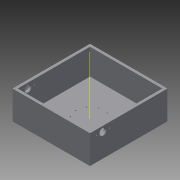
# Autodesk Inventor part: locomotion box
Saved by Autodesk Inventor 2015 (Build 190159000, 159)
## iProperties
Created: 2014-10-11
Part Number: locomotion box
Material: Generic
Document SubType Name: Modeling
Designer: ericd_000
Density: 1 g/cm^3
Appearance: Default
Author: ericd_000
Autodesk Inventor part; units mm, degrees
ref_plane "YZ Plane" through (0, 0, 0) normal (1, 0, 0) x (0, 1, 0)
ref_plane "XZ Plane" through (0, 0, 0) normal (0, 1, 0) x (-1, 0, 0)
ref_plane "XY Plane" through (0, 0, 0) normal (0, 0, 1) x (1, 0, 0)
sketch "Sketch1" plane through (0, 0, 0) normal (0, 0, 1) x (1, 0, 0)
  line L0 (-150, 150) -> (150, 150)
  line L1 (150, 150) -> (150, -150)
  line L2 (150, -150) -> (-150, -150)
  line L3 (-150, -150) -> (-150, 150)
  point P0 (0, 0)
  point P1 (150, 0)
  point P2 (0, 150)
  dimension "d0" = 300
  dimension "d1" = 300
  constraints: 8 end point, 2 midpoint, 2 parallel, 1 horizontal, 1 horizontal alignment, 1 perpendicular, 1 vertical alignment
  measures "d0" distance of L0.start L0.end
  measures "d1" distance of L0.end L1.end
extrude "Extrusion1" add sketch "Sketch1" along normal blind 10
sketch "Sketch2" plane through (0, 0, 10) normal (0, 0, 1) x (1, 0, 0)
  line L0 (-150, 150) -> (150, 150)
  line L1 (150, 150) -> (150, -150)
  line L2 (150, -150) -> (-150, -150)
  line L3 (-150, -150) -> (-150, 150)
  line L4 (140, 140) -> (-140, 140)
  line L5 (-140, 140) -> (-140, -140)
  line L6 (-140, -140) -> (140, -140)
  line L7 (140, -140) -> (140, 140)
  point P0 (0, 0)
  dimension "d4" = 10
  constraints: 16 end point, 4 parallel, 2 perpendicular, 1 horizontal, 3 other
  measures "d4" distance between parallel lines of L3 L5
extrude "Extrusion2" add sketch "Sketch2" along normal blind 100
sketch "Sketch3" plane through (-150, -150, 0) normal (-1, 0, 0) x (0, 0, 1)
  circle A0 centre (60, 250) radius 12.5
  circle A1 centre (90, 50) radius 13.3073
  line L0 (0, 300) -> (110, 300) projected
  line L1 (0, 0) -> (110, 0) projected
  line L2 (110, 300) -> (110, 0) projected
  point P0 (0, 150)
  dimension "d7" = 25
  dimension "d8" = 50
  dimension "d9" = 50
  dimension "d10" = 20
  dimension "d11" = 50
  constraints: 2 centre point
  measures "d7" diameter of A0
  measures "d8" distance from line of L0 A0.centre
  measures "d9" distance from line of L1 A1.centre
  measures "d10" distance from line of L2 A1.centre
  measures "d11" distance from line of L2 A0.centre
sketch "Sketch6" plane through (0, 0, 0) normal (0, 0, -1) x (-1, 0, 0)
  circle A0 centre (0, 0) radius 59.25
  dimension "d21" = 118.5
  constraints: 1 centre point, 1 coincident
  measures "d21" diameter of A0
extrude "Extrusion6" cut sketch "Sketch6" against normal blind 5
sketch "Sketch7" plane through (0, 0, 5) normal (0, 0, -1) x (-1, 0, 0)
  circle A0 centre (42.997, -32.6689) radius 2
  line L0 (42.997, -32.6689) -> (0, 0) construction
  dimension "d24" = 54
  dimension "d25" = 4
  constraints: 2 end point, 1 centre point
  measures "d24" distance of L0.start L0.end
  measures "d25" diameter of A0
extrude "Extrusion7" cut sketch "Sketch7" against normal up to surface (5 mm away)
pattern_circular "Circular Pattern1" count 10 over 360 about axis through (0, 0, 5) along (0, 0, 1) of "Extrusion7"
extrude "Extrusion8" cut sketch "Sketch3" against normal blind 10 contours A1
sketch "Sketch8" plane through (-150, -150, 0) normal (-1, 0, 0) x (0, 0, 1)
  circle A0 centre (90, 75.4) radius 2.05
  circle A1 centre (90, 24.6) radius 2.05
  line L0 (90, 24.6) -> (90, 75.4) construction
  line L1 (0, 0) -> (0, 300) construction
  circle A2 centre (90, 50) radius 13.3073 construction
  circle A3 centre (90, 50) radius 13.3073 construction
  point P0 (0, 150)
  dimension "d33" = 4.1
  dimension "d34" = 4.1
  dimension "d35" = 50.8
  dimension "d37" = 0
  constraints: 3 centre point, 2 end point, 1 coincident, 1 concentric, 1 midpoint, 1 parallel
  measures "d33" diameter of A0
  measures "d34" diameter of A1
  measures "d35" distance of L0.end L0.start
  measures "d37" radial gap between concentric circles of A2 A3
extrude "Extrusion9" cut sketch "Sketch8" against normal blind 10
mirror "Mirror2" about plane through (0, 0, 0) normal (1, 0, 0) of "Extrusion8", "Extrusion9"
body "Solid1"
